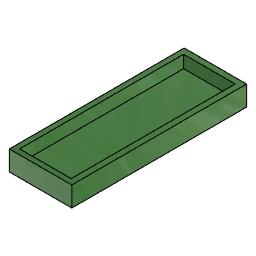
TofuGreenModel v1 (Autodesk Fusion 360 design; units mm, degrees)
Autodesk Fusion 360 part; units mm, degrees
sketch "Sketch1" plane through (0, 0, 0) normal (0, 0, 1) x (1, 0, 0)
  line L0 (-26.0373, -33.6026) -> (-1.0373, -33.6026)
  line L1 (-1.0373, -33.6026) -> (-1.0373, 36.3974)
  line L2 (-1.0373, 36.3974) -> (-26.0373, 36.3974)
  line L3 (-26.0373, 36.3974) -> (-26.0373, -33.6026)
  dimension "d1" = 25
  dimension "d2" = 70
  constraint horizontal L0
  constraint vertical L1
  constraint horizontal L2
  constraint vertical L3
  measures "d1" distance of L0.start L0.end
  measures "d2" distance of L0.start L2.end
extrude "Extrude1" add sketch "Sketch1" along normal blind 3
extrude "Extrude2" add 1 faces at (-17.7039, 13.0641, 3) along direction (0, 0, 1) blind 5
sketch "Sketch2" plane through (0, 0, 8) normal (0, 0, 1) x (-1, 0, 0)
  line L0 (26.0373, -36.3974) -> (26.0373, 33.6026)
  line L1 (26.0373, 33.6026) -> (1.0373, 33.6026)
  line L2 (1.0373, 33.6026) -> (1.0373, -36.3974)
  line L3 (1.0373, -36.3974) -> (26.0373, -36.3974)
  line L4 (23.98, -34.1191) -> (3.337, -34.1191)
  line L5 (3.337, -34.1191) -> (3.337, 31.543)
  line L6 (3.337, 31.543) -> (23.98, 31.543)
  line L7 (23.98, 31.543) -> (23.98, -34.1191)
  constraint horizontal L4
  constraint vertical L5
  constraint horizontal L6
  constraint vertical L7
extrude "Extrude3" cut sketch "Sketch2" against normal blind 5 contours L4 L5 L6 L7
